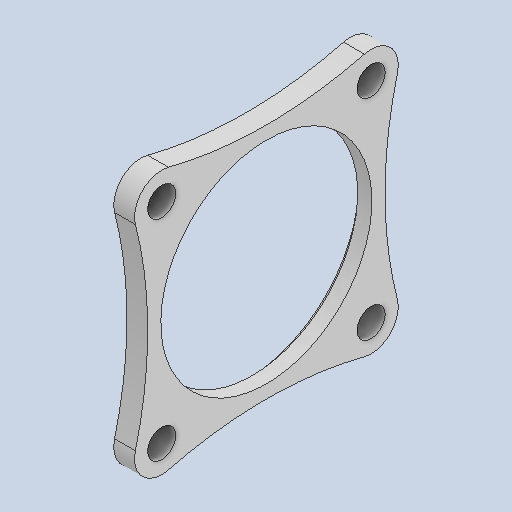
# Autodesk Inventor part: bearing older plate
Saved by Autodesk Inventor 2023 (Build 270158000, 158)
## iProperties
Created: 2022-08-31
Part Number: bearing older plate
Material: Generic
Document SubType Name: Modeling
Designer: deli
Density: 1 g/cm^3
Appearance: Default
Author: deli
Autodesk Inventor part; units mm, degrees
ref_plane "YZ Plane" through (0, 0, 0) normal (1, 0, 0) x (0, 1, 0)
ref_plane "XZ Plane" through (0, 0, 0) normal (0, 1, 0) x (-1, 0, 0)
ref_plane "XY Plane" through (0, 0, 0) normal (0, 0, 1) x (1, 0, 0)
sketch "Sketch1" plane through (0, 0, 0) normal (1, 0, 0) x (0, 1, 0)
  line L0 (105.4415, 125.8106) -> (114.0501, 137.6593) projected
  arc A0 (114.9535, 140.4398) -> (114.0501, 137.6593) centre (114.9535, 138.9028) ccw projected
  line L1 (114.9535, 140.4398) -> (114.9535, 155.0856) projected
  arc A1 (114.0501, 157.866) -> (114.9535, 155.0856) centre (114.9535, 156.6226) ccw projected
  line L2 (114.0501, 157.866) -> (105.4415, 169.7147) projected
  arc A2 (103.0763, 171.4331) -> (105.4415, 169.7147) centre (104.5381, 170.9582) ccw projected
  line L3 (103.0763, 171.4331) -> (89.1473, 175.9589) projected
  arc A3 (86.2238, 175.9589) -> (89.1473, 175.9589) centre (87.6856, 176.4339) ccw projected
  line L4 (86.2238, 175.9589) -> (72.2948, 171.4331) projected
  arc A4 (69.9296, 169.7147) -> (72.2948, 171.4331) centre (70.833, 170.9582) ccw projected
  line L5 (69.9296, 169.7147) -> (61.321, 157.866) projected
  arc A5 (60.4176, 155.0856) -> (61.321, 157.866) centre (60.4176, 156.6226) ccw projected
  line L6 (60.4176, 155.0856) -> (60.4176, 140.4398) projected
  arc A6 (61.321, 137.6593) -> (60.4176, 140.4398) centre (60.4176, 138.9028) ccw projected
  line L7 (61.321, 137.6593) -> (69.9296, 125.8106) projected
  arc A7 (72.2948, 124.0922) -> (69.9296, 125.8106) centre (70.833, 124.5672) ccw projected
  line L8 (72.2948, 124.0922) -> (86.2238, 119.5664) projected
  arc A8 (89.1473, 119.5664) -> (86.2238, 119.5664) centre (87.6856, 119.0915) ccw projected
  line L9 (89.1473, 119.5664) -> (103.0763, 124.0922) projected
  arc A9 (105.4415, 125.8106) -> (103.0763, 124.0922) centre (104.5381, 124.5672) ccw projected
  arc A10 (69.7246, 158.8833) -> (67.1217, 152.5995) centre (87.6856, 147.7627) ccw projected
  arc A11 (71.5859, 159.889) -> (69.7246, 158.8833) centre (71.5313, 157.7647) ccw projected
  arc A12 (71.5859, 159.889) -> (75.5593, 163.8623) centre (71.6856, 163.7627) ccw projected
  arc A13 (76.5649, 165.7237) -> (75.5593, 163.8623) centre (77.6836, 163.9169) ccw projected
  arc A14 (82.8487, 168.3265) -> (76.5649, 165.7237) centre (87.6856, 147.7627) ccw projected
  arc A15 (84.876, 167.7214) -> (82.8487, 168.3265) centre (83.3352, 166.2579) ccw projected
  arc A16 (84.876, 167.7214) -> (90.4951, 167.7214) centre (87.6856, 170.3901) ccw projected
  arc A17 (92.5224, 168.3265) -> (90.4951, 167.7214) centre (92.0359, 166.2579) ccw projected
  arc A18 (98.8062, 165.7237) -> (92.5224, 168.3265) centre (87.6856, 147.7627) ccw projected
  arc A19 (99.8118, 163.8623) -> (98.8062, 165.7237) centre (97.6875, 163.9169) ccw projected
  arc A20 (99.8118, 163.8623) -> (103.7852, 159.889) centre (103.6856, 163.7627) ccw projected
  arc A21 (105.6466, 158.8833) -> (103.7852, 159.889) centre (103.8398, 157.7647) ccw projected
  arc A22 (108.2494, 152.5995) -> (105.6466, 158.8833) centre (87.6856, 147.7627) ccw projected
  arc A23 (107.6443, 150.5723) -> (108.2494, 152.5995) centre (106.1808, 152.113) ccw projected
  arc A24 (107.6443, 150.5723) -> (107.6443, 144.9531) centre (110.313, 147.7627) ccw projected
  arc A25 (108.2494, 142.9258) -> (107.6443, 144.9531) centre (106.1808, 143.4124) ccw projected
  arc A26 (105.6466, 136.642) -> (108.2494, 142.9258) centre (87.6856, 147.7627) ccw projected
  arc A27 (103.7852, 135.6364) -> (105.6466, 136.642) centre (103.8398, 137.7607) ccw projected
  arc A28 (103.7852, 135.6364) -> (99.8118, 131.663) centre (103.6856, 131.7627) ccw projected
  arc A29 (98.8062, 129.8017) -> (99.8118, 131.663) centre (97.6875, 131.6084) ccw projected
  arc A30 (92.5224, 127.1989) -> (98.8062, 129.8017) centre (87.6856, 147.7627) ccw projected
  arc A31 (90.4951, 127.8039) -> (92.5224, 127.1989) centre (92.0359, 129.2674) ccw projected
  arc A32 (90.4951, 127.8039) -> (84.876, 127.8039) centre (87.6856, 125.1353) ccw projected
  arc A33 (82.8487, 127.1989) -> (84.876, 127.8039) centre (83.3352, 129.2674) ccw projected
  arc A34 (76.5649, 129.8017) -> (82.8487, 127.1989) centre (87.6856, 147.7627) ccw projected
  arc A35 (75.5593, 131.663) -> (76.5649, 129.8017) centre (77.6836, 131.6084) ccw projected
  arc A36 (75.5593, 131.663) -> (71.5859, 135.6364) centre (71.6856, 131.7627) ccw projected
  arc A37 (69.7246, 136.642) -> (71.5859, 135.6364) centre (71.5313, 137.7607) ccw projected
  arc A38 (67.1217, 142.9258) -> (69.7246, 136.642) centre (87.6856, 147.7627) ccw projected
  arc A39 (67.7268, 144.9531) -> (67.1217, 142.9258) centre (69.1903, 143.4124) ccw projected
  arc A40 (67.7268, 144.9531) -> (67.7268, 150.5723) centre (65.0581, 147.7627) ccw projected
  arc A41 (67.1217, 152.5995) -> (67.7268, 150.5723) centre (69.1903, 152.113) ccw projected
  circle A42 centre (110.313, 147.7627) radius 2.15 projected
  circle A43 centre (103.6856, 131.7627) radius 2.15 projected
  circle A44 centre (103.6856, 163.7627) radius 2.15 projected
  circle A45 centre (87.6856, 170.3901) radius 2.15 projected
  circle A46 centre (71.6856, 163.7627) radius 2.15 projected
  circle A47 centre (65.0581, 147.7627) radius 2.15 projected
  circle A48 centre (71.6856, 131.7627) radius 2.15 projected
  circle A49 centre (87.6856, 125.1353) radius 2.15 projected
  circle A50 centre (87.6856, 147.7627) radius 16 construction
  circle A51 centre (87.6856, 147.7627) radius 16.125
  circle A52 centre (87.6856, 147.7627) radius 18.125 construction
  arc A53 (102.6517, 127.7435) -> (107.7047, 132.7966) centre (103.6856, 131.7627) ccw
  arc A54 (107.7047, 162.7288) -> (102.6517, 167.7818) centre (103.6856, 163.7627) ccw
  arc A55 (67.6664, 132.7966) -> (72.7195, 127.7435) centre (71.6856, 131.7627) ccw
  arc A56 (72.7195, 167.7818) -> (67.6664, 162.7288) centre (71.6856, 163.7627) ccw
  arc A57 (107.7047, 162.7288) -> (107.7047, 132.7966) centre (165.8829, 147.7627) ccw
  arc A58 (102.6517, 127.7435) -> (72.7195, 127.7435) centre (87.6856, 69.5653) ccw
  arc A59 (67.6664, 132.7966) -> (67.6664, 162.7288) centre (9.4882, 147.7627) ccw
  arc A60 (72.7195, 167.7818) -> (102.6517, 167.7818) centre (87.6856, 225.9601) ccw
  point P0 (0, 0)
  dimension "d0" = 32
  dimension "d1" = 0.125
  dimension "d2" = 2
  dimension "d3" = 2
  dimension "d4" = 2
  dimension "d5" = 2
  dimension "d6" = 2
  constraints: 16 point on circle, 12 tangent, 11 centre point, 3 coincident
  measures "d0" diameter of A50
  measures "d1" radial gap between concentric circles of A50 A51
  measures "d2" radial gap between concentric circles of A51 A52
  measures "d3" radial gap between concentric circles of A43 A53
  measures "d4" radial gap between concentric circles of A44 A54
  measures "d5" radial gap between concentric circles of A55 A48
  measures "d6" radial gap between concentric circles of A56 A46
extrude "Extrusion1" add sketch "Sketch1" along normal blind 3.175 contours A11 A12 A13 A14 A60 A18 A19 A20 A21 A22 A57 A26 A27 A28 A29 A30 A58 A34 A35 A36 A37 A38 A59 A10 | A10 A59 A56 A60 A14 A13 A12 A11 | A38 A37 A36 A35 A34 A58 A55 A59 | A60 A54 A57 A22 A21 A20 A19 A18 | A30 A29 A28 A27 A26 A57 A53 A58
sketch "Sketch2" plane through (0, 0, 0) normal (-1, 0, 0) x (0, 0, 1)
  circle A0 centre (147.7627, 87.6856) radius 16.125 projected
  circle A1 centre (147.7627, 87.6856) radius 17.25
  point P0 (0, 0)
  dimension "d11" = 34.5
  constraints: 1 centre point, 1 coincident
  measures "d11" diameter of A1
extrude "Extrusion2" cut sketch "Sketch2" against normal blind 1
equation "\"d4\" = d3"
body "Solid1"
